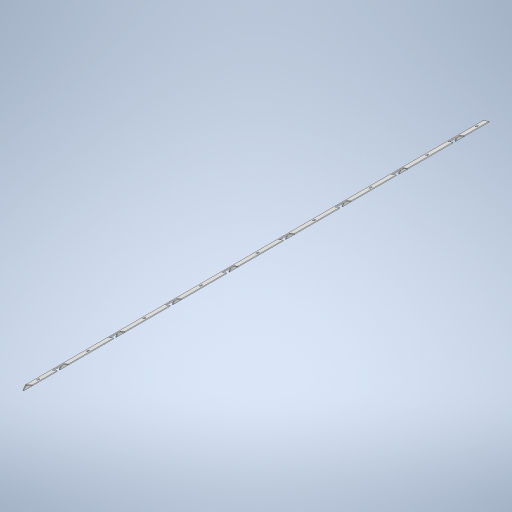
# Autodesk Inventor part: ДМС 103 Полка для крышки
Saved by Autodesk Inventor 2024.2 (Build 282272000, 272)
## iProperties
Created: 2024-04-30
Part Number: ДМС 103 Полка для крышки
Material: Generic
Document SubType Name: Sheet Metal
Designer: pokla
Density: 1 g/cm^3
Appearance: Default
Sheet Metal Rule: Default
Author: pokla
Autodesk Inventor part; units mm, degrees
ref_plane "YZ Plane" through (0, 0, 0) normal (1, 0, 0) x (0, 1, 0)
ref_plane "XZ Plane" through (0, 0, 0) normal (0, 1, 0) x (-1, 0, 0)
ref_plane "XY Plane" through (0, 0, 0) normal (0, 0, 1) x (1, 0, 0)
sketch "Sketch4" plane through (0, 0, 0) normal (0, 0, 1) x (1, 0, 0)
  line L0 (-193.637817, 193.637817) -> (0, 273.845227) construction
  line L1 (0, 273.845227) -> (193.637817, 193.637817) construction
  line L2 (193.637817, 193.637817) -> (273.845227, 0) construction
  line L3 (273.845227, 0) -> (193.637817, -193.637817) construction
  line L4 (193.637817, -193.637817) -> (0, -273.845227) construction
  line L5 (0, -273.845227) -> (-193.637817, -193.637817) construction
  line L6 (-193.637817, -193.637817) -> (-273.845227, 0) construction
  line L7 (-273.845227, 0) -> (-193.637817, 193.637817) construction
  line L8 (-191.341716, 191.341716) -> (0, 270.59805) construction
  line L9 (0, 270.59805) -> (191.341716, 191.341716) construction
  line L10 (191.341716, 191.341716) -> (270.59805, 0) construction
  line L11 (270.59805, 0) -> (191.341716, -191.341716) construction
  line L12 (191.341716, -191.341716) -> (0, -270.59805) construction
  line L13 (0, -270.59805) -> (-191.341716, -191.341716) construction
  line L14 (-191.341716, -191.341716) -> (-270.59805, 0) construction
  line L15 (-270.59805, 0) -> (-191.341716, 191.341716) construction
  line L16 (-189.045616, 192.292792) -> (-162.715049, 203.19927)
  line L17 (-192.292792, 189.045616) -> (-203.19927, 162.715049)
  arc A0 (-189.045616, 192.292792) -> (-192.292792, 189.045616) centre (-186.749515, 186.749515) ccw
  point P0 (0, 0)
  point P1 (0, 0)
  point P2 (0, 0)
  dimension "d16" = 506
  dimension "d22" = 3
  dimension "d23" = 28.5
  dimension "d24" = 6
  measures "d16" distance between parallel lines of L7 L3
  measures "d22" distance between parallel lines of L7 L15
  measures "d23" distance of L16.start L16.end
  measures "d24" radius of A0
contour flange "Contour Flange1" sketch "Sketch4" thickness 3 bend radius 3 width 2020 along (0, 0, -1) mid plane no both sides no wall seen from (-175.880332, 197.746031, 0) lies toward (0.3826834, -0.9238795, 0) curves L16 A0 L17
bend "Bend2"
corner "Corner2"
sketch "Sketch6" plane through (-189.045616, 192.292792, 0) normal (-0.3826834, 0.9238795, 0) x (0.9238795, 0.3826834, 0)
  circle A0 centre (14.25, 40.75) radius 5.5
  line L0 (28.5, 0) -> (0, 0) projected
  circle A1 centre (14.25, 1979.25) radius 5.5
  line L1 (28.5, 2020) -> (0, 2020) projected
  point P0 (101.068109, 0)
  point P1 (14.25, 0)
  point P2 (14.25, 0)
  point P3 (14.25, 0)
  point P4 (14.25, 0)
  point P5 (14.25, 2020)
  point P6 (14.25, 2020)
  dimension "d36" = 11
  dimension "d37" = 40.75
  dimension "d40" = 40.75
  dimension "d41" = 11
  constraints: 6 midpoint, 2 centre point, 2 vertical alignment
  measures "d36" diameter of A0
  measures "d37" distance of point (14.25, 0) A0.centre
  measures "d40" distance of point (14.25, 2020) A1.centre
  measures "d41" diameter of A1
extrude "Extrusion1" cut sketch "Sketch6" against normal up to surface (3 mm away)
sketch "Sketch10" plane through (-189.045616, 192.292792, 0) normal (-0.3826834, 0.9238795, 0) x (0.9238795, 0.3826834, 0)
  line L0 (6.5, 1160) -> (28.5, 1160)
  line L1 (28.5, 1160) -> (28.5, 1110)
  line L2 (28.5, 1110) -> (6.5, 1110)
  line L3 (6.5, 1110) -> (6.5, 1160)
  line L4 (28.5, 2020) -> (0, 2020) projected
  line L5 (0, 0) -> (0, 2020) projected
  point P0 (0, 1010)
  point P1 (6.5, 1135)
  dimension "d70" = 50
  dimension "d71" = 22
  dimension "d72" = 125
  constraints: 8 end point, 2 midpoint, 2 parallel, 1 horizontal, 1 perpendicular, 1 vertical alignment
  measures "d70" distance of L0.end L1.end
  measures "d71" distance of L1.end L2.end
  measures "d72" vertical distance of point (0, 1010) point (6.5, 1135)
extrude "Extrusion5" cut sketch "Sketch10" against normal through all
sketch "Sketch12" plane through (-192.292792, 189.045616, -2020) normal (-0.9238795, 0.3826834, 0) x (0, 0, 1)
  line L0 (860, -28.5) -> (910, -28.5)
  line L1 (910, -28.5) -> (910, -6.5)
  line L2 (910, -6.5) -> (860, -6.5)
  line L3 (860, -6.5) -> (860, -28.5)
  line L4 (2020, 0) -> (0, 0) projected
  point P0 (2020, -101.068109)
  point P1 (0, -28.5)
  point P2 (1010, 0)
  point P3 (885, -6.5)
  dimension "d75" = 50
  dimension "d76" = 22
  dimension "d77" = 125
  constraints: 8 end point, 2 midpoint, 2 parallel, 1 horizontal, 1 horizontal alignment, 1 perpendicular
  measures "d75" distance of L0.start L0.end
  measures "d76" distance of L2.end L0.start
  measures "d77" horizontal distance of point (1010, 0) point (885, -6.5)
extrude "Extrusion6" cut sketch "Sketch12" against normal through all
pattern_linear "Rectangular Pattern4" count 8 spacing 250 along (0, 0, 1) of "Extrusion6", "Extrusion5" first direction both ways yes
sketch "Sketch13" plane through (-189.045616, 192.292792, 0) normal (-0.3826834, 0.9238795, 0) x (0.9238795, 0.3826834, 0)
  circle A0 centre (14.25, 1010) radius 5.5
  line L0 (28.5, 910) -> (28.5, 1110) projected
  line L1 (28.5, 0) -> (0, 0) projected
  point P0 (101.068109, 0)
  point P1 (28.5, 1010)
  point P2 (14.25, 0)
  dimension "d83" = 11
  constraints: 2 midpoint, 1 centre point, 1 horizontal alignment, 1 vertical alignment
  measures "d83" diameter of A0
extrude "Extrusion7" cut sketch "Sketch13" against normal through all
pattern_linear "Rectangular Pattern5" count 7 spacing 250 along (0, 0, 1) of "Extrusion7" first direction both ways yes
equation "\"d40\" = d37"
equation "\"d72\" = Отступ_окна_от_середины"
equation "\"d77\" = Отступ_окна_от_середины"
equation "\"d16\" = Барабан_габарит_по_кассетам"
equation "\"d24\" = BendRadius + Thickness"
equation "\"d41\" = d36"
equation "\"d70\" = Ширина_окна_барабан"
equation "\"d75\" = Ширина_окна_барабан"
equation "\"d25\" = Thickness"
equation "\"d26\" = BendReliefWidth"
equation "\"d27\" = BendReliefDepth"
equation "\"d28\" = MinimumRemnant"
equation "\"d29\" = TransitionRadius"
equation "\"d30\" = Барабан_длина_листа"
equation "\"d31\" = BendRadius"
equation "\"d33\" = CornerReliefSize"
equation "\"d34\" = GapSize"
equation "\"d35\" = JacobiRadiusSize"
equation "\"BendRadius\" = Thickness"
equation "\"BendReliefWidth\" = Thickness"
equation "\"BendReliefDepth\" = 0.5 * Thickness"
equation "\"CornerReliefSize\" = 4 * Thickness"
equation "\"MinimumRemnant\" = 2 * Thickness"
equation "\"TransitionRadius\" = BendRadius"
equation "\"JacobiRadiusSize\" = BendRadius"
equation "\"GapSize\" = Thickness"
equation "\"Барабан_габарит_по_кассетам\" = 506"
equation "\"Thickness\" = 3"
equation "\"Ширина_окна_барабан\" = 50"
equation "\"Барабан_длина_листа\" = 2020"
equation "\"Отступ_окна_от_середины\" = 125"
body "Solid2"
